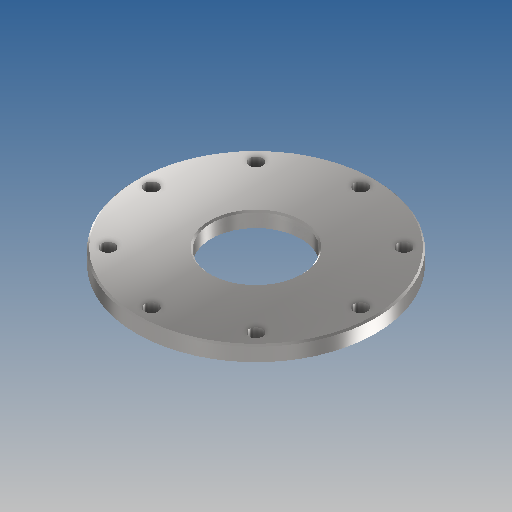
# Autodesk Inventor part: PWTR-0070
Saved by Autodesk Inventor 2021.1 (Build 251245000, 245)
## iProperties
Created: 2020-08-28
Part Number: PWTR-0070
Material: Stainless Steel
Document SubType Name: Modeling
Designer: alid
Density: 8 g/cm^3
Appearance: Semi-Polished
Description: Input Shaft Access Bonnet
Author: alid
Revision Number: A
Autodesk Inventor part; units mm, degrees
ref_plane "YZ Plane" through (0, 0, 0) normal (1, 0, 0) x (0, 1, 0)
ref_plane "XZ Plane" through (0, 0, 0) normal (0, 1, 0) x (-1, 0, 0)
ref_plane "XY Plane" through (0, 0, 0) normal (0, 0, 1) x (1, 0, 0)
sketch "Sketch1" plane through (0, 0, 0) normal (0, 0, 1) x (1, 0, 0)
  circle A0 centre (0, 0) radius 40
  circle A1 centre (0, 0) radius 15
  circle A2 centre (0, 0) radius 35 construction
  line L0 (0, 0) -> (0, 35) construction
  line L1 (0, 0) -> (13.3939, 32.3358) construction
  dimension "d0" = 80
  dimension "d1" = 30
  dimension "d2" = 70
  dimension "d3" = 22.5
  constraints: 4 end point, 3 centre point, 3 coincident, 2 point on circle, 1 vertical
  measures "d0" diameter of A0
  measures "d1" diameter of A1
  measures "d2" diameter of A2
  measures "d3" angle of L1 L0
extrude "Extrusion1" add sketch "Sketch1" along normal blind 5
hole "Hole1" at (0, 35, 0) direction (0, 0, 1) diameter 4.5 depth 11.8 clearance for "Socket Head Cap Screw ISO 4762" size "M4" standard "ISO"
pattern_circular "Circular Pattern1" count 8 over 360 about axis through (0, 0, -10) along (0, 0, 1) of "Hole1"
chamfer "Chamfer1" distance 0.5 angle 45 2 edges at (-40, 0, 5) (-15, 0, 5)
body "Solid1"
